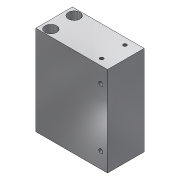
# Autodesk Inventor part: BC-10015
Saved by Autodesk Inventor 2016 (Build 200138000, 138)
## iProperties
Created: 2015-11-06
Part Number: BC-10015
Project: DIPOLO BC-3T- SIRIUS
Cost Center: 1504002005
Material: Alumínio 7075
Document SubType Name: Modeling
Designer: reinaldo.basilio
Density: 2.81 g/cm^3
Appearance: Aluminum - Polished
Mass: 1078.33 g
Surface Area: 442.649 cm^2
Volume: 383.748 cm^3
Description: Posicionador dos blocos magnéticos na lateral.
RuleStatus: InUse
AfterMaterialChange0: file://_iMaterial
AfterAnyiPropertyChange0: file://_iMaterial
AfterDocNew0: file://_Naming_par
AfterDocNew1: file://_NameStart
AfterDocNew2: file://_NameStart1
AfterDocNew3: file://_Materiais
DocNumber: XXXXX-XXX-XXXX-00-001.ipt
Folder: .
Title: DIPOLO BC-3T- SIRIUS
Author: reinaldo.basilio
Subject: BC-10015
Autodesk Inventor part; units mm, degrees
ref_plane "YZ Plane" through (0, 0, 0) normal (1, 0, 0) x (0, 1, 0)
ref_plane "XZ Plane" through (0, 0, 0) normal (0, 1, 0) x (-1, 0, 0)
ref_plane "XY Plane" through (0, 0, 0) normal (0, 0, 1) x (1, 0, 0)
sketch "Sketch5" plane through (0, 0, 0) normal (0, 0, 1) x (1, 0, 0)
  line L0 (-22, 43) -> (22, 43)
  line L1 (22, 43) -> (22, -43)
  line L2 (22, -43) -> (-22, -43)
  line L3 (-22, -43) -> (-22, 43)
  point P0 (0, 0)
  point P1 (22, 0)
  point P2 (0, 43)
  dimension "d8" = 86
  dimension "d9" = 44
  constraints: 8 end point, 2 midpoint, 2 parallel, 1 horizontal, 1 horizontal alignment, 1 perpendicular, 1 vertical alignment
  measures "d8" distance of L2.end L0.start
  measures "d9" distance of L0.start L0.end
extrude "Extrusion5" add sketch "Sketch5" along normal mid plane 107.5
sketch "Sketch6" plane through (0, 0, 53.75) normal (0, 0, 1) x (1, 0, 0)
  line L0 (22, 43) -> (-22, 43) projected
  circle A0 centre (14, -33) radius 4
  circle A1 centre (-14, -33) radius 4
  circle A2 centre (-14, -33) radius 8.5
  point P0 (0, 0)
  dimension "d12" = 76
  dimension "d13" = 28
  dimension "d14" = 14
  dimension "d15" = 8
  dimension "d17" = 17
  constraints: 3 centre point, 1 coincident, 1 equal radius, 1 horizontal alignment
  measures "d12" distance from line of A0.centre L0
  measures "d13" distance of A1.centre A0.centre
  measures "d14" horizontal distance of point (0, 0) A0.centre
  measures "d15" diameter of A0
  measures "d17" diameter of A2
hole "Hole1" at (-14, -33, 53.75) at (14, -33, 53.75) direction (0, 0, -1) diameter 8.5 end through all counterbore diameter 14 counterbore depth 45 clearance for "Socket Head Cap Screw DIN EN ISO 4762" size "M8" standard "DIN"
sketch "Sketch7" plane through (22, -43, 53.75) normal (1, 0, 0) x (0, 0, -1)
  line L0 (0, 86) -> (107.5, 86) projected
  circle A0 centre (18.75, 78) radius 3
  circle A1 centre (88.75, 78) radius 3
  point P0 (53.75, 43)
  dimension "d25" = 8
  dimension "d26" = 70
  dimension "d27" = 35
  dimension "d28" = 6
  dimension "d45" = 107.5
  dimension "d46" = 18.75
  constraints: 2 centre point, 1 equal radius, 1 horizontal alignment
  measures "d25" distance from line of L0 A0.centre
  measures "d26" distance of A0.centre A1.centre
  measures "d27" horizontal distance of point (53.75, 43) A0.centre
  measures "d28" diameter of A0
  measures "d45" distance of L0.start L0.end
  measures "d46" horizontal distance of A0.centre L0.start
hole "Hole2" at (22, 35, 35) at (22, 35, -35) direction (-1, 0, 0) diameter 4.917 end through all thread size "M6x1" class "6H" standard "ANSI Metric M Profile"
sketch "Sketch8" plane through (0, 0, 53.75) normal (0, 0, 1) x (1, 0, 0)
  circle A0 centre (-14, -33) radius 7 projected
  circle A1 centre (14, -33) radius 7 projected
  line L0 (22, 43) -> (-22, 43) projected
  circle A2 centre (14, 28) radius 4
  circle A3 centre (-14, 28) radius 4
  point P0 (0, 0)
  dimension "d36" = 15
  dimension "d37" = 8
  constraints: 2 centre point, 2 vertical alignment, 1 equal radius, 1 horizontal alignment
  measures "d36" distance from line of A3.centre L0
  measures "d37" diameter of A2
hole "Hole3" at (-14, 28, 53.75) at (14, 28, 53.75) direction (0, 0, -1) diameter 4.134 depth 15 tip angle 118 thread size "M5x0.8" class "6H" standard "ANSI Metric M Profile"
equation "\"d14\" = 0.5 * d13"
equation "\"d27\" = 0.5 * d26"
body "Solid5"
